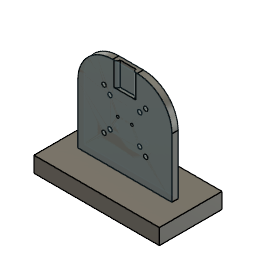
suporte_motor_COM_case_encoder (Autodesk Fusion 360 design; units mm, degrees)
Autodesk Fusion 360 part; units mm, degrees
sketch "Esboço1" plane through (0, 0, 0) normal (0, 0, 1) x (1, 0, 0)
  line L0 (-30, 0) -> (-30, 7.8)
  line L1 (-7.8, 30) -> (7.8, 30)
  line L2 (30, 7.8) -> (30, -30)
  line L3 (30, -30) -> (-30, -30)
  line L4 (-30, -30) -> (-30, 0)
  line L5 (0, -30) -> (40, -30)
  line L6 (40, -30) -> (40, -40)
  line L7 (40, -40) -> (-40, -40)
  line L8 (-40, -40) -> (-40, -30)
  line L9 (-30, -30) -> (-40, -30)
  circle A0 centre (0, 0) radius 4
  circle A1 centre (9.5, 9.5) radius 1.35
  circle A2 centre (-9.5, 9.5) radius 1.35
  circle A3 centre (-9.5, -9.5) radius 1.35
  circle A4 centre (9.5, -9.5) radius 1.35
  arc A5 (-7.8, 30) -> (-30, 7.8) centre (-7.8, 7.8) ccw
  arc A6 (30, 7.8) -> (7.8, 30) centre (7.8, 7.8) ccw
  point P0 (-30, 30)
  point P1 (30, 30)
  dimension "d3" = 60
  dimension "d4" = 60
  dimension "d7" = 10
  dimension "d8" = 80
  dimension "d13" = 8
  dimension "d16" = 2.7
  dimension "d18" = 360
  dimension "d28" = 22.2
  dimension "d29" = 22.2
  constraint perpendicular L0 L1
  constraint perpendicular L1 L2
  constraint perpendicular L2 L3
  constraint midpoint L3 L5.start
  constraint perpendicular L2 L5
  constraint perpendicular L5 L6
  constraint perpendicular L6 L7
  constraint perpendicular L7 L8
  constraint perpendicular L8 L9
  constraint coincident A0.centre origin
  constraint coincident P0 L1
  constraint coincident P0 L0
  constraint tangent L1 A5
  constraint tangent L0 A5
  constraint coincident P1 L1
  constraint coincident P1 L2
  constraint tangent L1 A6
  constraint tangent L2 A6
  measures "d3" distance of P0 P1
  measures "d4" distance of P1 L2.end
  measures "d7" distance of L5.end L6.end
  measures "d8" distance of L6.end L7.end
  measures "d13" diameter of A0
  measures "d16" diameter of A1
  measures "d28" radius of A5
  measures "d29" radius of A6
extrude "Extrusão1" add sketch "Esboço1" along normal mid plane 40 contours L3 L5 L6 L7 L8 L9
extrude "Extrusão2" add sketch "Esboço1" along normal mid plane 4 contours L0 L1 L2 L3 L4 L5 A5 A6 | A0 | A1 | A2 | A3 | A4
ref_plane "Plano de trabalho1" through (0, 0, 2) normal (0, 0, 1) x (1, 0, 0)
sketch "Esboço2" plane through (0, 0, 2) normal (0, 0, 1) x (1, 0, 0)
  circle A0 centre (0, 0) radius 4
  circle A1 centre (9.5, 9.5) radius 1.35
  circle A2 centre (-9.5, 9.5) radius 1.35
  circle A3 centre (-9.5, -9.5) radius 1.35
  circle A4 centre (9.5, -9.5) radius 1.35
  dimension "d20" = 8
  dimension "d23" = 2.7
  dimension "d25" = 360
  constraint coincident A0.centre origin
  measures "d20" diameter of A0
  measures "d23" diameter of A1
extrude "Extrusão3" cut sketch "Esboço2" against normal blind 21 contours A1 | A2 | A3 | A4
ref_plane "Plano de trabalho2" through (0, -30, 0) normal (0, 1, 0) x (-1, 0, 0)
sketch "Esboço3" plane through (0, -30, 0) normal (0, 1, 0) x (1, 0, 0)
sketch "Esboço4" plane through (0, 0, -2) normal (0, 0, -1) x (-1, 0, 0)
  circle A0 centre (9.5, 9.5) radius 1.35
  circle A1 centre (9.5, -9.5) radius 1.35
  circle A2 centre (-9.5, 9.5) radius 1.35
  circle A3 centre (-9.5, -9.5) radius 1.35
  line L0 (-30, -30) -> (30, -30)
  line L1 (30, -30) -> (30, 7.8)
  arc A4 (30, 7.8) -> (7.8, 30) centre (7.8, 7.8) ccw
  line L2 (7.8, 30) -> (-7.8, 30)
  arc A5 (-7.8, 30) -> (-30, 7.8) centre (-7.8, 7.8) ccw
  line L3 (-30, 7.8) -> (-30, -30)
sketch "Esboço5" plane through (0, 0, 2) normal (0, 0, 1) x (1, 0, 0)
  circle A0 centre (-9.5, 9.5) radius 1.35
  circle A1 centre (-9.5, -9.5) radius 1.35
  circle A2 centre (9.5, 9.5) radius 1.35
  circle A3 centre (9.5, -9.5) radius 1.35
  line L0 (-30, -30) -> (30, -30)
  line L1 (30, -30) -> (30, 7.8)
  arc A4 (30, 7.8) -> (7.8, 30) centre (7.8, 7.8) ccw
  line L2 (7.8, 30) -> (-7.8, 30)
  arc A5 (-7.8, 30) -> (-30, 7.8) centre (-7.8, 7.8) ccw
  line L3 (-30, 7.8) -> (-30, -30)
sketch "Esboço6" plane through (0, 0, 2) normal (0, 0, 1) x (1, 0, 0)
sketch "Esboço7" plane through (0, 0, 2) normal (0, 0, 1) x (1, 0, 0)
  circle A0 centre (13.3, 13.3) radius 1.35
  circle A1 centre (-13.3, 13.3) radius 1.35
  circle A2 centre (-13.3, -13.3) radius 1.35
  circle A3 centre (13.3, -13.3) radius 1.35
  dimension "d34" = 2.7
  dimension "d36" = 360
  measures "d34" diameter of A0
extrude "Extrusão5" cut sketch "Esboço7" against normal blind 18
sketch "Esboço8" plane through (0, 0, 2) normal (0, 0, 1) x (1, 0, 0)
  circle A0 centre (-4.5, 0) radius 0.8
  circle A1 centre (4.5, 0) radius 0.8
  dimension "d39" = 1.6
  dimension "d40" = 1.6
  measures "d39" diameter of A0
  measures "d40" diameter of A1
extrude "Extrusão6" cut sketch "Esboço8" against normal blind 25
sketch "Esboço9" plane through (0, 30, 0) normal (0, 1, 0) x (-1, 0, 0)
  line L0 (7.8, -2) -> (7.8, 2)
  line L1 (7.8, 2) -> (-7.8, 2)
  line L2 (-7.8, 2) -> (-7.8, -2)
  line L3 (-7.8, -2) -> (7.8, -2)
  line L4 (5, 2) -> (5, 0)
  line L5 (5, 0) -> (-5, 0)
  line L6 (-5, 0) -> (-5, 2)
  line L7 (5, 2) -> (-5, 2)
  line L8 (-5, 2) -> (5, 2)
  constraint coincident L1 L4.start
  constraint perpendicular L1 L4
  constraint perpendicular L4 L5
  constraint coincident L1 L6.end
  constraint perpendicular L1 L6
extrude "Extrusão7" cut sketch "Esboço9" against normal blind 15 contours L1 L4 L5 L6 L7 L8
fillet "Arredondamento1" radius 2 2 edges at (5, 22.5, 2) (-5, 22.5, 2)
